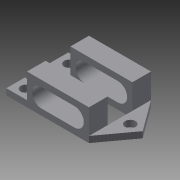
# Autodesk Inventor part: push_clip(1)
Saved by Autodesk Inventor 2015 (Build 190159000, 159)
## iProperties
Created: 2017-10-04
Part Number: push_clip(1)
Material: Generic
Document SubType Name: Modeling
Designer: Anshul
Density: 1 g/cm^3
Appearance: Default
Author: Anshul
Autodesk Inventor part; units mm, degrees
ref_plane "YZ Plane" through (0, 0, 0) normal (1, 0, 0) x (0, 1, 0)
ref_plane "XZ Plane" through (0, 0, 0) normal (0, 1, 0) x (-1, 0, 0)
ref_plane "XY Plane" through (0, 0, 0) normal (0, 0, 1) x (1, 0, 0)
sketch "Sketch1" plane through (0, 0, 0) normal (0, 1, 0) x (-1, 0, 0)
  circle A0 centre (0, 0) radius 3.2
  circle A1 centre (0, 0) radius 3.4
  circle A2 centre (0, 0) radius 5
  circle A3 centre (0, 0) radius 6
  line L0 (0, 0) -> (0, -15)
  line L1 (0, 0) -> (0, 15)
  line L2 (0, 0) -> (-9, 0)
  circle A4 centre (-9, 0) radius 3.75
  line L3 (0, 15) -> (0, 6)
  line L4 (0, 6) -> (10, 6)
  line L5 (10, 6) -> (10, 15)
  line L6 (10, 15) -> (0, 15)
  line L7 (10, 10.5) -> (5, 10.5)
  line L8 (0, -15) -> (10, -15)
  line L9 (10, -15) -> (10, -6)
  line L10 (10, -6) -> (0, -6)
  line L11 (10, -10.5) -> (5, -10.5)
  circle A5 centre (5, 10.5) radius 2.5
  circle A6 centre (5, -10.5) radius 2.5
  line L12 (0, -6) -> (-30, -6)
  line L13 (-30, -6) -> (-30, 6)
  line L14 (-30, 6) -> (0, 6)
  line L15 (0, 15) -> (-30, 15)
  line L16 (-30, 15) -> (-30, 6)
  line L17 (0, -15) -> (-30, -15)
  line L18 (-30, -15) -> (-30, -6)
  line L19 (-35, 0) -> (-41, 0)
  line L20 (-41, 0) -> (-30, -15)
  line L21 (-41, 0) -> (-30, 15)
  circle A7 centre (-35, 0) radius 2.5
  dimension "d3" = 12
  dimension "d0" = 6.4
  dimension "d1" = 6.8
  dimension "d2" = 10
  dimension "d4" = 15
  dimension "d5" = 15
  dimension "d6" = 9
  dimension "d7" = 7.5
  dimension "d8" = 10
  dimension "d9" = 5
  dimension "d10" = 10
  dimension "d11" = 10
  dimension "d12" = 5
  dimension "d13" = 5
  dimension "d14" = 5
  dimension "d15" = 30
  dimension "d17" = 6
  dimension "d18" = 5
  constraints: 44 end point, 8 coincident, 7 centre point, 7 horizontal, 7 perpendicular, 5 point on line, 2 midpoint, 2 vertical, 1 parallel, 1 vertical alignment, 2 other
  measures "d0" diameter of A0
  measures "d1" diameter of A1
  measures "d2" diameter of A2
  measures "d4" distance of L0.start L0.end
  measures "d5" distance of L0.start L1.end
  measures "d6" distance of L0.start L2.end
  measures "d7" diameter of A4
  measures "d8" distance of L3.end L4.end
  measures "d9" distance of L7.start L7.end
  measures "d10" distance of L0.end L8.end
  measures "d11" distance of L9.end L10.end
  measures "d12" distance of L11.start L11.end
  measures "d13" diameter of A5
  measures "d14" diameter of A6
  measures "d15" distance of L10.end L12.end
  measures "d17" distance of L19.start L19.end
  measures "d18" diameter of A7
extrude "Extrusion1" add sketch "Sketch1" along normal blind 3 contours L1 L6 L5 L4 | L10 L9 L8 L0 | L13 L18 L20 L21 L16
extrude "Extrusion2" add sketch "Sketch1" along normal blind 15 contours L14 L16 L15 L1 | L0 L17 L18 L12
sketch "Sketch2" plane through (-10, 0, 15) normal (0, 0, 1) x (1, 0, 0)
  line L0 (10, 15) -> (10, 7.5)
  line L1 (10, 3) -> (10, 15) projected
  line L2 (10, 7.5) -> (17, 7.5)
  arc A0 (17, 12) -> (17, 3) centre (17, 7.5) ccw
  line L3 (17, 7.5) -> (40, 7.5)
  line L4 (40, 3) -> (40, 15) projected
  line L5 (40, 7.5) -> (33, 7.5)
  arc A1 (33, 3) -> (33, 12) centre (33, 7.5) ccw
  line L6 (17, 3) -> (33, 3)
  line L7 (17, 12) -> (33, 12)
  point P0 (10, 0)
  dimension "d23" = 7.5
  dimension "d24" = 7
  dimension "d25" = 9
  dimension "d26" = 7
  dimension "d27" = 9
  constraints: 12 end point, 4 point on circle, 3 point on line, 2 centre point, 2 coincident, 2 horizontal, 2 tangent
  measures "d23" distance of L0.start L0.end
  measures "d24" distance of L0.end L2.end
  measures "d25" diameter of A0
  measures "d26" distance of L3.end L5.end
  measures "d27" diameter of A1
extrude "Extrusion3" cut sketch "Sketch2" against normal blind 31
body "Solid1"
